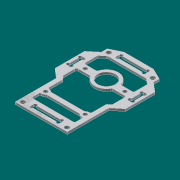
# Autodesk Inventor part: 胴体_サブフレーム_1_11
Saved by Autodesk Inventor 2016 (Build 200138000, 138)
## iProperties
Created: 2016-05-21
Part Number: 胴体_サブフレーム_1_11
Material: アルミニウム 2014-T4
Document SubType Name: Modeling
Designer: hiroaki
Density: 2.8 g/cm^3
Appearance: サテン
Mass: 4.59557 g
Surface Area: 33.0865 cm^2
Volume: 1.64127 cm^3
Author: hiroaki
Autodesk Inventor part; units mm, degrees
ref_plane "YZ Plane" through (0, 0, 0) normal (1, 0, 0) x (0, 1, 0)
ref_plane "XZ Plane" through (0, 0, 0) normal (0, 1, 0) x (-1, 0, 0)
ref_plane "XY Plane" through (0, 0, 0) normal (0, 0, 1) x (1, 0, 0)
derived "胴体_基礎_1_5.ipt"
sketch "スケッチ1" plane through (0, 0, 0) normal (0, 0, 1) x (1, 0, 0)
  circle A0 centre (0, 0) radius 11 construction
  line L0 (-10, 19) -> (10, 19) construction
  line L1 (10, 19) -> (10, 16.5) construction
  line L2 (10, 16.5) -> (-10, 16.5) construction
  line L3 (-10, 16.5) -> (-10, 19) construction
  line L4 (-10, -39.5) -> (10, -39.5) construction
  line L5 (10, -39.5) -> (10, -42) construction
  line L6 (10, -42) -> (-10, -42) construction
  line L7 (-10, -42) -> (-10, -39.5) construction
  line L8 (0, 0) -> (0, 19) construction
  line L9 (-10.583, 12) -> (10.583, 12) construction
  arc A1 (-10.583, 12) -> (-16, 0) centre (0, 0) ccw construction
  line L10 (-16, 0) -> (-16, -39.5) construction
  line L11 (-16, -39.5) -> (16, -39.5) construction
  line L12 (16, -39.5) -> (16, 0) construction
  arc A2 (16, 0) -> (10.583, 12) centre (0, 0) ccw construction
  line L13 (-13.5, -1) -> (13.5, -1) construction
  line L14 (13.5, -1) -> (13.5, -28) construction
  line L15 (13.5, -28) -> (-13.5, -28) construction
  line L16 (-13.5, -28) -> (-13.5, -1) construction
  circle A3 centre (-13.5, -1) radius 1.35
  circle A4 centre (-13.5, -28) radius 1.35
  circle A5 centre (13.5, -28) radius 1.35
  circle A6 centre (13.5, -1) radius 1.35
  circle A7 centre (-15, 16.5) radius 1.55
  circle A8 centre (15, 16.5) radius 1.55
  circle A9 centre (-15, -42) radius 1.55
  circle A10 centre (15, -42) radius 1.55
  line L17 (0, 19) -> (0, -42) construction
  line L18 (-15, -42) -> (15, -42) construction
  line L19 (15, -42) -> (15, 16.5) construction
  line L20 (15, 16.5) -> (-15, 16.5) construction
  line L21 (-15, 16.5) -> (-15, -42) construction
  line L22 (-15, -42) -> (15, 16.5) construction
  line L23 (15, -42) -> (-15, 16.5) construction
  circle A11 centre (-15, 16.5) radius 2.75 construction
  line L24 (-17.75, 18.218) -> (-17.75, -44.5) construction
  line L25 (-17.75, -44.5) -> (-10, -44.5)
  line L26 (-10, -44.5) -> (10, -44.5)
  line L27 (10, -44.5) -> (17.75, -44.5)
  line L28 (17.75, -44.5) -> (17.75, 18.218) construction
  line L29 (17.75, 18.218) -> (10, 22)
  line L30 (10, 22) -> (-10, 22)
  line L31 (-10, 22) -> (-17.75, 18.218)
  line L32 (10.05, 19.05) -> (-10.05, 19.05)
  line L33 (-10.05, 19.05) -> (-10.05, 16.45)
  line L34 (-10.05, 16.45) -> (10.05, 16.45)
  line L35 (10.05, 16.45) -> (10.05, 19.05)
  circle A12 centre (-9, 19.05) radius 1.05
  circle A13 centre (-9, 16.45) radius 1.05
  circle A14 centre (9, 19.05) radius 1.05
  circle A15 centre (9, 16.45) radius 1.05
  line L36 (-10.05, -39.45) -> (10.05, -39.45)
  line L37 (10.05, -39.45) -> (10.05, -42.05)
  line L38 (10.05, -42.05) -> (-10.05, -42.05)
  line L39 (-10.05, -42.05) -> (-10.05, -39.45)
  circle A16 centre (-9, -39.45) radius 1.05
  circle A17 centre (-9, -42.05) radius 1.05
  circle A18 centre (9, -39.45) radius 1.05
  circle A19 centre (9, -42.05) radius 1.05
  line L40 (-22, 5) -> (-20, 5) construction
  line L41 (-20, 5) -> (-20, -5) construction
  line L42 (-20, -5) -> (-22, -5) construction
  line L43 (-22, -5) -> (-22, 5) construction
  line L44 (20, 5) -> (22, 5) construction
  line L45 (22, 5) -> (22, -5) construction
  line L46 (22, -5) -> (20, -5) construction
  line L47 (20, -5) -> (20, 5) construction
  line L48 (-17.75, 18.218) -> (-17.75, 14.2444)
  line L49 (-17.75, 14.2444) -> (-24, 9)
  line L50 (-24, 9) -> (-24, -11)
  line L51 (-24, -11) -> (-17.75, -16.2444)
  line L52 (-17.75, -16.2444) -> (-17.75, -44.5)
  line L53 (17.75, 18.218) -> (17.75, 14.2444)
  line L54 (17.75, 14.2444) -> (24, 9)
  line L55 (24, 9) -> (24, -11)
  line L56 (24, -11) -> (17.75, -16.2444)
  line L57 (17.75, -16.2444) -> (17.75, -44.5)
  line L58 (-19.9, 5.1) -> (-22.1, 5.1)
  line L59 (-22.1, 5.1) -> (-22.1, -5.1)
  line L60 (-22.1, -5.1) -> (-19.9, -5.1)
  line L61 (-19.9, -5.1) -> (-19.9, 5.1)
  line L62 (19.9, 5.1) -> (22.1, 5.1)
  line L63 (22.1, 5.1) -> (22.1, -5.1)
  line L64 (22.1, -5.1) -> (19.9, -5.1)
  line L65 (19.9, -5.1) -> (19.9, 5.1)
  circle A20 centre (-22.1, 4.05) radius 1.05
  circle A21 centre (-19.9, 4.05) radius 1.05
  circle A22 centre (-19.9, -4.05) radius 1.05
  circle A23 centre (-22.1, -4.05) radius 1.05
  circle A24 centre (19.9, 4.05) radius 1.05
  circle A25 centre (22.1, 4.05) radius 1.05
  circle A26 centre (22.1, -4.05) radius 1.05
  circle A27 centre (19.9, -4.05) radius 1.05
  circle A28 centre (0, 0) radius 6.05
  circle A29 centre (-15, -42) radius 2.75 construction
  point P0 (0, -1)
  point P1 (-10, 16.5)
  point P2 (-22, 0)
  dimension "d1" = 12.1
  measures "d1" diameter of A28
extrude "押し出し1" add sketch "スケッチ1" along normal blind 1.5
sketch "スケッチ3" plane through (-17.75, -44.5, 1.5) normal (0, 0, 1) x (1, 0, 0)
  line L0 (25.7, 2.45) -> (9.8, 2.45) projected
  arc A0 (7.7, 2.45) -> (9.8, 2.45) centre (8.75, 2.45) ccw projected
  line L1 (7.7, 2.45) -> (7.7, 5.05) projected
  arc A1 (9.8, 5.05) -> (7.7, 5.05) centre (8.75, 5.05) ccw projected
  line L2 (9.8, 5.05) -> (25.7, 5.05) projected
  arc A2 (27.8, 5.05) -> (25.7, 5.05) centre (26.75, 5.05) ccw projected
  line L3 (27.8, 5.05) -> (27.8, 2.45) projected
  arc A3 (25.7, 2.45) -> (27.8, 2.45) centre (26.75, 2.45) ccw projected
  circle A4 centre (17.75, 44.5) radius 6.05 projected
  line L4 (-2.15, 39.4) -> (-4.35, 39.4) projected
  arc A5 (-4.35, 41.5) -> (-4.35, 39.4) centre (-4.35, 40.45) ccw projected
  line L5 (-4.35, 41.5) -> (-4.35, 47.5) projected
  arc A6 (-4.35, 49.6) -> (-4.35, 47.5) centre (-4.35, 48.55) ccw projected
  line L6 (-4.35, 49.6) -> (-2.15, 49.6) projected
  arc A7 (-2.15, 47.5) -> (-2.15, 49.6) centre (-2.15, 48.55) ccw projected
  line L7 (-2.15, 47.5) -> (-2.15, 41.5) projected
  arc A8 (-2.15, 39.4) -> (-2.15, 41.5) centre (-2.15, 40.45) ccw projected
  circle A9 centre (31.25, 16.5) radius 1.35 projected
  circle A10 centre (4.25, 16.5) radius 1.35 projected
  circle A11 centre (4.25, 43.5) radius 1.35 projected
  circle A12 centre (2.75, 61) radius 1.55 projected
  line L8 (0, 58.7444) -> (-6.25, 53.5) projected
  line L9 (-6.25, 33.5) -> (0, 28.2556) projected
  line L10 (0, 28.2556) -> (0, 0) projected
  line L11 (3, 29.6546) -> (3, 18.6651)
  line L12 (6.25, 18) -> (29.25, 18)
  line L13 (32.5, 18.6651) -> (32.5, 29.6546)
  arc A13 (6.25, 18) -> (3, 18.6651) centre (4.25, 16.5) ccw
  line L14 (3, 29.6546) -> (0.8, 31.5006)
  line L15 (0.8, 31.5006) -> (0.8, 41)
  line L16 (0.8, 41) -> (10.5007, 41)
  line L17 (-2.15, 49.55) -> (-4.35, 49.55) construction
  arc A14 (-4.35, 49.55) -> (-4.3, 47.5513) centre (-4.35, 48.55) ccw construction
  line L18 (-4.3, 47.5513) -> (-4.3, 41.4487) construction
  arc A15 (-4.3, 41.4487) -> (-4.35, 39.45) centre (-4.35, 40.45) ccw construction
  line L19 (-4.35, 39.45) -> (-2.15, 39.45) construction
  arc A16 (-2.15, 39.45) -> (-2.2, 41.4487) centre (-2.15, 40.45) ccw construction
  line L20 (-2.2, 41.4487) -> (-2.2, 47.5513) construction
  arc A17 (-2.2, 47.5513) -> (-2.15, 49.55) centre (-2.15, 48.55) ccw construction
  arc A18 (10.5007, 41) -> (24.9993, 41) centre (17.75, 44.5) ccw
  line L21 (24.9993, 41) -> (34.7, 41)
  line L22 (34.7, 41) -> (34.7, 31.5006)
  line L23 (34.7, 31.5006) -> (32.5, 29.6546)
  line L24 (17.75, 44.5) -> (17.75, 50.55) construction
  arc A19 (32.5, 18.6651) -> (29.25, 18) centre (31.25, 16.5) ccw
  line L25 (17.75, 44.5) -> (11.7, 44.5) construction
  line L26 (4.3759, 58.5) -> (31.1241, 58.5)
  line L27 (0.8, 55.4994) -> (4.3759, 58.5)
  line L28 (31.1241, 58.5) -> (34.7, 55.4994)
  line L29 (0.8, 55.4994) -> (0.8, 46)
  line L30 (0.8, 46) -> (9.841, 46)
  line L31 (34.7, 55.4994) -> (34.7, 46)
  line L32 (34.7, 46) -> (25.659, 46)
  arc A20 (25.659, 46) -> (9.841, 46) centre (17.75, 44.5) ccw
  line L33 (3, 14.3349) -> (3, 8)
  line L34 (3, 8) -> (32.5, 8)
  line L35 (32.5, 8) -> (32.5, 14.3349)
  arc A21 (3, 14.3349) -> (6.25, 15) centre (4.25, 16.5) ccw
  line L36 (6.25, 15) -> (29.25, 15)
  arc A22 (29.25, 15) -> (32.5, 14.3349) centre (31.25, 16.5) ccw
  line L37 (25.7513, 5) -> (9.7487, 5) construction
  arc A23 (9.7487, 5) -> (7.75, 5.05) centre (8.75, 5.05) ccw construction
  line L38 (7.75, 5.05) -> (7.75, 2.45) construction
  arc A24 (7.75, 2.45) -> (9.7487, 2.5) centre (8.75, 2.45) ccw construction
  line L39 (9.7487, 2.5) -> (25.7513, 2.5) construction
  arc A25 (25.7513, 2.5) -> (27.75, 2.45) centre (26.75, 2.45) ccw construction
  line L40 (27.75, 2.45) -> (27.75, 5.05) construction
  arc A26 (27.75, 5.05) -> (25.7513, 5) centre (26.75, 5.05) ccw construction
  dimension "d4" = 2.5
  dimension "d5" = 3
  dimension "d6" = 1.5
  dimension "d7" = 2.5
  dimension "d8" = 0.05
  dimension "d9" = 3
  dimension "d10" = 3
  dimension "d11" = 2
  dimension "d12" = 2.5
  dimension "d13" = 3
  dimension "d14" = 2.5
  dimension "d15" = 1.5
  dimension "d16" = 0.05
  dimension "d17" = 3
  constraints: 60 end point, 30 point on circle, 14 centre point, 7 vertical, 6 coincident, 6 horizontal, 5 perpendicular, 4 equal radius, 4 symmetric about line, 3 vertical alignment, 2 horizontal alignment, 2 parallel, 15 other
  measures "d4" radius of A13
  measures "d5" distance between parallel lines of L10 L11
  measures "d6" distance from line of A13.centre L12
  measures "d7" distance from line of A11.centre L16
  measures "d8" radial gap between concentric circles of A7 A17
  measures "d9" distance between parallel lines of L15 L20
  measures "d10" distance between parallel lines of L14 L9
  measures "d11" radial gap between concentric circles of A18 A4
  measures "d12" distance from line of L26 A12.centre
  measures "d13" distance between parallel lines of L27 L8
  measures "d14" distance from line of A11.centre L30
  measures "d15" distance from line of L36 A10.centre
  measures "d16" distance between parallel lines of L2 L37
  measures "d17" distance between parallel lines of L37 L34
extrude "押し出し2" cut sketch "スケッチ3" against normal blind 1.5 contours L14 L15 L16 A18 L21 L22 L23 L13 A19 L12 A13 L11 | L26 L28 L31 L32 A20 L30 L29 L27 | A21 L36 A22 L35 L34 L33
fillet "フィレット1" radius 1.05 26 edges at (-16.95, -3.5, 0.75) (-7.2493, -3.5, 0.75) (-16.95, 1.5, 0.75) (-16.95, 10.9994, 0.75) (-13.3741, 14, 0.75) (13.3741, 14, 0.75) (16.95, 10.9994, 0.75) (16.95, 1.5, 0.75) (16.95, -3.5, 0.75) (7.2493, -3.5, 0.75) (7.909, 1.5, 0.75) (-7.909, 1.5, 0.75) (-14.75, -14.8454, 0.75) (-16.95, -12.9994, 0.75) (-14.75, -30.1651, 0.75) (-14.75, -36.5, 0.75) (-11.5, -29.5, 0.75) (-11.5, -26.5, 0.75) (-14.75, -25.8349, 0.75) (14.75, -36.5, 0.75) (14.75, -30.1651, 0.75) (11.5, -29.5, 0.75) (16.95, -12.9994, 0.75) (14.75, -14.8454, 0.75) (14.75, -25.8349, 0.75) (11.5, -26.5, 0.75)
equation "\"d6\" = 0.5 * d5"
equation "\"d7\" = d4"
equation "\"d9\" = d5"
equation "\"d10\" = d5"
equation "\"d13\" = d10"
equation "\"d14\" = d7"
equation "\"d15\" = d6"
